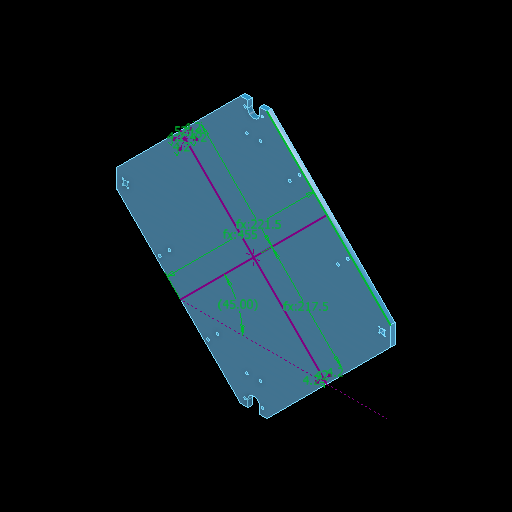
# Autodesk Inventor part: z_plate
Saved by Autodesk Inventor 2026.1 (Build 301233000, 233)
## iProperties
Created: 2025-09-21
Part Number: z_plate
Material: Aluminum 6061
Document SubType Name: Modeling
Designer: drago
Density: 2.7 g/cm^3
Appearance: Sky Blue Dark
Mass: 5370.18 g
Surface Area: 4188.49 cm^2
Volume: 1988.96 cm^3
Author: drago
Autodesk Inventor part; units mm, degrees
ref_plane "YZ Plane" through (0, 0, 0) normal (1, 0, 0) x (0, 1, 0)
ref_plane "XZ Plane" through (0, 0, 0) normal (0, 1, 0) x (-1, 0, 0)
ref_plane "XY Plane" through (0, 0, 0) normal (0, 0, 1) x (1, 0, 0)
sketch "Sketch2" plane through (0, 0, 0) normal (0, 0, 1) x (1, 0, 0)
  circle A0 centre (0, 277.5) radius 8 construction
  circle A1 centre (0, 277.5) radius 13
  circle A2 centre (0, 277.5) radius 10.5 construction
  line L0 (25, 287.5) -> (-25, 287.5) construction
  line L1 (-25, 287.5) -> (-25, 222.5) construction
  line L2 (-25, 222.5) -> (25, 222.5) construction
  line L3 (25, 222.5) -> (25, 287.5) construction
  circle A3 centre (15, 228.5) radius 2.7
  circle A4 centre (-15, 228.5) radius 2.7
  circle A5 centre (-19, 277.5) radius 2.7
  circle A6 centre (19, 277.5) radius 2.7
  circle A7 centre (0, -277.5) radius 8 construction
  circle A8 centre (0, -277.5) radius 13
  circle A9 centre (0, -277.5) radius 10.5 construction
  line L4 (25, -287.5) -> (-25, -287.5) construction
  line L5 (-25, -287.5) -> (-25, -222.5) construction
  line L6 (-25, -222.5) -> (25, -222.5) construction
  line L7 (25, -222.5) -> (25, -287.5) construction
  circle A10 centre (-15, -228.5) radius 2.7
  circle A11 centre (15, -228.5) radius 2.7
  circle A12 centre (-19, -277.5) radius 2.7
  circle A13 centre (19, -277.5) radius 2.7
  line L8 (10.5, -277.5) -> (10.5, -287.5) construction
  line L9 (-10.5, -277.5) -> (-10.5, -287.5) construction
  line L10 (10.5, 277.5) -> (10.5, 287.5) construction
  line L11 (-10.5, 277.5) -> (-10.5, 287.5) construction
  circle A14 centre (281.7, 0) radius 5.25
  circle A15 centre (-281.7, 0) radius 5.25
  line L12 (0, -321.7336) -> (321.7336, 0)
  line L13 (321.7336, 0) -> (0, 321.7336)
  line L14 (0, 321.7336) -> (-321.7336, 0)
  line L15 (-321.7336, 0) -> (0, -321.7336)
  line L16 (0, -321.7336) -> (0, 321.7336) construction
  line L17 (321.7336, 0) -> (-321.7336, 0) construction
  line L18 (0, -321.7336) -> (455, -321.7336) construction
  line L19 (300.5, 21.2336) -> (300.5, -21.2336)
  line L20 (-300.5, 21.2336) -> (-300.5, -21.2336)
  line L21 (-24.2336, 297.5) -> (24.2336, 297.5) construction
  line L22 (-29.2336, 292.5) -> (29.2336, 292.5)
  line L23 (-24.2336, -297.5) -> (24.2336, -297.5) construction
  line L24 (-29.2336, -292.5) -> (29.2336, -292.5)
  line L25 (-9.5, 297.5) -> (-3.976, 284.442) construction
  line L26 (9.5, 297.5) -> (3.976, 284.442) construction
  line L27 (-14.929, 297.5) -> (-9.9883, 285.8207)
  line L28 (14.929, 297.5) -> (9.9883, 285.8207)
  line L29 (-9.5, -297.5) -> (-3.976, -284.442) construction
  line L30 (9.5, -297.5) -> (3.976, -284.442) construction
  line L31 (14.929, -297.5) -> (9.9883, -285.8207)
  line L32 (-14.929, -297.5) -> (-9.9883, -285.8207)
  line L33 (13, 277.5) -> (13, 292.5)
  line L34 (-13, 277.5) -> (-13, 292.5)
  line L35 (-13, -277.5) -> (-13, -292.5)
  line L36 (13, -277.5) -> (13, -292.5)
  line L37 (281.7, 0) -> (287.3569, 5.6569) construction
  line L38 (281.7, 0) -> (289.7, 0) construction
  circle A16 centre (287.3569, 5.6569) radius 1.6
  circle A17 centre (276.0431, 5.6569) radius 1.6
  circle A18 centre (276.0431, -5.6569) radius 1.6
  circle A19 centre (287.3569, -5.6569) radius 1.6
  line L39 (-281.7, 0) -> (-287.3569, 5.6569) construction
  circle A20 centre (-287.3569, 5.6569) radius 1.6
  circle A21 centre (-287.3569, -5.6569) radius 1.6
  circle A22 centre (-276.0431, -5.6569) radius 1.6
  circle A23 centre (-276.0431, 5.6569) radius 1.6
  point P0 (0, 0)
  point P1 (-12.8138, -292.5)
  point P2 (12.8138, -292.5)
  point P3 (12.8138, 292.5)
  point P4 (-12.8138, 292.5)
  point P5 (300.5, 292.5)
  point P6 (300.5, -292.5)
  point P7 (-300.5, -292.5)
  point P8 (-300.5, 292.5)
  dimension "d349" = 450
  dimension "d350" = 45
  dimension "d353" = 40
  dimension "d354" = 10
  dimension "d355" = 10
  dimension "d358" = 40
  dimension "d359" = 10
  dimension "d360" = 10
  dimension "d361" = 6.2
  dimension "d362" = 75
  dimension "d363" = 5
  dimension "d364" = 6.2
  dimension "d365" = 5
  dimension "d366" = 75
  dimension "d367" = 450
  dimension "d368" = 45
  dimension "d369" = 6.2
  dimension "d370" = 5
  dimension "d371" = 75
  dimension "d372" = 6.2
  dimension "d373" = 5
  dimension "d374" = 75
  dimension "d256" = 16
  dimension "d257" = 0
  dimension "d258" = 277.5
  dimension "d259" = 26
  dimension "d260" = 21
  dimension "d261" = 50
  dimension "d262" = 10
  dimension "d263" = 65
  dimension "d265" = 50
  dimension "d266" = 25
  dimension "d267" = 5.4
  dimension "d268" = 5.4
  dimension "d269" = 5.4
  dimension "d270" = 5.4
  dimension "d271" = 6
  dimension "d272" = 10
  dimension "d273" = 6
  dimension "d274" = 10
  dimension "d275" = 6
  dimension "d276" = 10
  dimension "d277" = 6
  dimension "d278" = 10
  dimension "d279" = 0
  dimension "d280" = 277.5
  dimension "d281" = 26
  dimension "d282" = 16
  dimension "d283" = 21
  dimension "d284" = 50
  dimension "d285" = 10
  dimension "d286" = 65
  dimension "d287" = 25
  dimension "d288" = 5.4
  dimension "d289" = 5.4
  dimension "d290" = 5.4
  dimension "d291" = 5.4
  dimension "d292" = 6
  dimension "d293" = 10
  dimension "d294" = 6
  dimension "d295" = 10
  dimension "d296" = 10
  dimension "d297" = 6
  dimension "d298" = 10
  dimension "d299" = 6
  dimension "d300" = 10.5
  dimension "d301" = 0
  dimension "d302" = 281.7
  dimension "d310" = 10.5
  dimension "d311" = 0
  dimension "d312" = 281.7
  dimension "d320" = 455
  dimension "d321" = 45
  dimension "d322" = 455
  dimension "d323" = 18.8
  dimension "d324" = 18.8
  dimension "d325" = 20
  dimension "d326" = 15
  dimension "d327" = 20
  dimension "d328" = 15
  dimension "d329" = 67.07
  dimension "d330" = 67.07
  dimension "d331" = 9.5
  dimension "d332" = 9.5
  dimension "d333" = 67.07
  dimension "d334" = 67.07
  constraints: 80 end point, 32 point on line, 24 centre point, 16 point on circle, 9 perpendicular, 7 horizontal, 6 coincident, 6 tangent, 4 parallel, 4 vertical, 2 equal length, 2 midpoint, 19 other
  measures "d256" diameter of A0
  measures "d257" horizontal distance of point (0, 0) A0.centre
  measures "d258" distance of point (0, 0) A0.centre
  measures "d259" diameter of A1
  measures "d260" diameter of A2
  measures "d261" distance of L0.start L0.end
  measures "d262" distance from line of A2.centre L0
  measures "d263" distance of L0.end L1.end
  measures "d265" distance of L1.end L2.end
  measures "d266" distance from line of A2.centre L1
  measures "d267" diameter of A3
  measures "d268" diameter of A4
  measures "d269" diameter of A5
  measures "d270" diameter of A6
  measures "d271" distance from line of L2 A3.centre
  measures "d272" distance from line of L3 A3.centre
  measures "d273" distance from line of L2 A4.centre
  measures "d274" distance from line of L1 A4.centre
  measures "d275" distance from line of L3 A6.centre
  measures "d276" distance from line of L0 A6.centre
  measures "d277" distance from line of L1 A5.centre
  measures "d278" distance from line of L0 A5.centre
  measures "d279" horizontal distance of point (0, 0) A8.centre
  measures "d280" distance of point (0, 0) A8.centre
  measures "d281" diameter of A8
  measures "d282" diameter of A7
  measures "d283" diameter of A9
  measures "d284" distance of L4.start L4.end
  measures "d285" distance from line of L4 A8.centre
  measures "d286" distance of L4.end L5.end
  measures "d287" distance from line of A8.centre L5
  measures "d288" diameter of A10
  measures "d289" diameter of A11
  measures "d290" diameter of A12
  measures "d291" diameter of A13
  measures "d292" distance from line of L6 A10.centre
  measures "d293" distance from line of L5 A10.centre
  measures "d294" distance from line of L6 A11.centre
  measures "d295" distance from line of L7 A11.centre
  measures "d296" distance from line of L4 A12.centre
  measures "d297" distance from line of L5 A12.centre
  measures "d298" distance from line of L4 A13.centre
  measures "d299" distance from line of L7 A13.centre
  measures "d300" diameter of A14
  measures "d301" vertical distance of L37.start point (0, 0)
  measures "d302" distance of point (0, 0) L37.start
  measures "d310" diameter of A15
  measures "d311" vertical distance of point (0, 0) L39.start
  measures "d312" distance of point (0, 0) L39.start
  measures "d320" distance of L12.start L12.end
  measures "d321" angle of L18 L12
  measures "d322" distance of L13.end L12.end
  measures "d323" distance from line of L19 L37.start
  measures "d324" distance from line of L39.start L20
  measures "d325" distance from line of A1.centre L21
  measures "d326" distance from line of A1.centre L22
  measures "d327" distance from line of L23 A8.centre
  measures "d328" distance from line of A8.centre L24
  measures "d329" angle of L21 L25
  measures "d330" angle of L26 L21
  measures "d331" horizontal distance of A1.centre L26.start
  measures "d332" horizontal distance of A1.centre L25.start
  measures "d333" angle of L27 L21
  measures "d334" angle of L28 L21
ref_plane "Work Plane1" through (0, 0, 0) normal (0, 0, 1) x (1, 0, 0)
sketch "Sketch3" plane through (0, 0, 0) normal (0, 0, 1) x (1, 0, 0)
  line L0 (-159.099, -159.099) -> (159.099, 159.099)
  line L1 (-159.099, -159.099) -> (290.901, -159.099) construction
  line L2 (279.2843, 34.9264) -> (34.9264, 279.2843)
  line L3 (34.9264, 279.2843) -> (6.6421, 251)
  line L4 (6.6421, 251) -> (251, 6.6421)
  line L5 (251, 6.6421) -> (279.2843, 34.9264)
  line L6 (279.2843, 34.9264) -> (6.6421, 251) construction
  line L7 (34.9264, 279.2843) -> (251, 6.6421) construction
  circle A0 centre (19, 277.5) radius 2.7 projected
  circle A1 centre (15, 228.5) radius 2.7 projected
  line L8 (-34.9264, -279.2843) -> (-279.2843, -34.9264)
  line L9 (-279.2843, -34.9264) -> (-251, -6.6421)
  line L10 (-251, -6.6421) -> (-6.6421, -251)
  line L11 (-6.6421, -251) -> (-34.9264, -279.2843)
  line L12 (-34.9264, -279.2843) -> (-251, -6.6421) construction
  line L13 (-279.2843, -34.9264) -> (-6.6421, -251) construction
  circle A2 centre (-15, -228.5) radius 2.7 projected
  circle A3 centre (-19, -277.5) radius 2.7 projected
  circle A4 centre (-79.3236, -185.3896) radius 3.1
  circle A5 centre (-100.5368, -206.6028) radius 3.1
  circle A6 centre (-185.3896, -79.3236) radius 3.1
  circle A7 centre (-206.6028, -100.5368) radius 3.1
  line L14 (-159.099, 159.099) -> (159.099, -159.099)
  line L15 (300.5, -21.2336) -> (29.2336, -292.5) projected
  line L16 (-159.099, 159.099) -> (290.901, 159.099) construction
  circle A8 centre (206.6028, 100.5368) radius 3.1
  circle A9 centre (185.3896, 79.3236) radius 3.1
  circle A10 centre (100.5368, 206.6028) radius 3.1
  circle A11 centre (79.3236, 185.3896) radius 3.1
  point P0 (0, 0)
  point P1 (142.9632, 142.9632)
  point P2 (-142.9632, -142.9632)
  point P3 (29.2336, -292.5)
  dimension "d349" = 450
  dimension "d350" = 45
  dimension "d353" = 40
  dimension "d354" = 10
  dimension "d355" = 10
  dimension "d358" = 40
  dimension "d359" = 10
  dimension "d360" = 10
  dimension "d361" = 6.2
  dimension "d362" = 75
  dimension "d363" = 5
  dimension "d364" = 6.2
  dimension "d365" = 5
  dimension "d366" = 75
  dimension "d367" = 450
  dimension "d368" = 45
  dimension "d369" = 6.2
  dimension "d370" = 5
  dimension "d371" = 75
  dimension "d372" = 6.2
  dimension "d373" = 5
  dimension "d374" = 75
  constraints: 32 end point, 8 centre point, 6 midpoint, 4 parallel, 4 perpendicular, 4 symmetric about line, 2 equal length, 2 horizontal, 2 point on line, 7 other
  measures "d349" distance of L0.start L0.end
  measures "d350" angle of L1 L0
  measures "d353" distance of L3.end L2.end
  measures "d354" distance from line of L3 A0.centre
  measures "d355" distance from line of A1.centre L4
  measures "d358" distance of L8.end L9.end
  measures "d359" distance from line of A2.centre L10
  measures "d360" distance from line of L11 A3.centre
  measures "d361" diameter of A4
  measures "d362" distance from line of L0 A4.centre
  measures "d363" distance from line of L10 A4.centre
  measures "d364" diameter of A5
  measures "d365" distance from line of L8 A5.centre
  measures "d366" distance from line of L0 A5.centre
  measures "d367" distance of L14.start L14.end
  measures "d368" angle of L14 L16
  measures "d369" diameter of A8
  measures "d370" distance from line of L2 A8.centre
  measures "d371" distance from line of L0 A8.centre
  measures "d372" diameter of A9
  measures "d373" distance from line of L4 A9.centre
  measures "d374" distance from line of L0 A9.centre
extrude "Extrusion12" add sketch "Sketch2" against normal blind 10 contours L33 L22 L13 L19 L12 L24 L36 A8 L35 L15 L20 L14 L34 A1
hole "Hole2" at (100.5368, 206.6028, 0) at (79.3236, 185.3896, 0) at (206.6028, 100.5368, 0) at (185.3896, 79.3236, 0) at (-79.3236, -185.3896, 0) at (-100.5368, -206.6028, 0) at (-185.3896, -79.3236, 0) at (-206.6028, -100.5368, 0) direction (0, 0, -1) diameter 6.2 end through all
sketch "Sketch4" plane through (0, 0, 0) normal (0, 0, 1) x (1, 0, 0)
  line L0 (-160.8668, -160.8668) -> (160.8668, 160.8668)
  line L1 (29.2336, 292.5) -> (300.5, 21.2336) projected
  line L2 (-160.8668, -160.8668) -> (294.1332, -160.8668) construction
  line L3 (160.8668, -160.8668) -> (-160.8668, 160.8668)
  line L4 (-175.0089, 138.2394) -> (-138.2394, 175.0089) construction
  line L5 (-138.2394, 175.0089) -> (-125.5115, 162.281) construction
  line L6 (-125.5115, 162.281) -> (-162.281, 125.5115) construction
  line L7 (-162.281, 125.5115) -> (-175.0089, 138.2394) construction
  line L8 (-175.0089, 138.2394) -> (-125.5115, 162.281) construction
  line L9 (-138.2394, 175.0089) -> (-162.281, 125.5115) construction
  circle A0 centre (-138.2394, 175.0089) radius 2.1
  circle A1 centre (-125.5115, 162.281) radius 2.1
  circle A2 centre (-175.0089, 138.2394) radius 2.1
  circle A3 centre (-162.281, 125.5115) radius 2.1
  circle A4 centre (138.9465, -168.645) radius 2.1
  circle A5 centre (168.645, -138.9465) radius 2.1
  line L10 (138.9465, -168.645) -> (168.645, -138.9465) construction
  point P0 (0, 0)
  point P1 (-150.2602, 150.2602)
  point P2 (153.7957, -153.7957)
  dimension "d406" = 455
  dimension "d407" = 45
  dimension "d413" = 52
  dimension "d415" = 18
  dimension "d416" = 221.5
  dimension "d417" = 4.2
  dimension "d418" = 4.2
  dimension "d419" = 4.2
  dimension "d420" = 4.2
  dimension "d421" = 4.2
  dimension "d422" = 4.2
  dimension "d423" = 42
  dimension "d424" = 217.5
  constraints: 20 end point, 6 centre point, 6 coincident, 5 midpoint, 5 perpendicular, 2 equal length, 2 parallel, 2 point on line, 1 horizontal, 1 other
  measures "d406" distance of L0.start L0.end
  measures "d407" angle of L2 L0
  measures "d413" distance of L4.start L4.end
  measures "d415" distance of L4.end L5.end
  measures "d416" distance between parallel lines of L0 L4
  measures "d417" diameter of A0
  measures "d418" diameter of A1
  measures "d419" diameter of A2
  measures "d420" diameter of A3
  measures "d421" diameter of A4
  measures "d422" diameter of A5
  measures "d423" distance of L10.start L10.end
  measures "d424" distance between parallel lines of L10 L0
equation "\"dist_rails\" = 555"
equation "\"dist_leadscrews\" = 563.4"
equation "\"diam_leadscrew_hole\" = 10.5"
equation "\"z_plate_width\" = 455"
equation "\"delta\" = 5"
equation "\"rail_angle\" = 67.07deg"
equation "\"rail_D\" = 9.5"
equation "\"rail_diam\" = 16"
body "Solid10"
